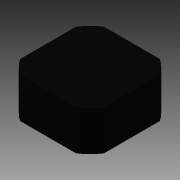
# Autodesk Inventor part: stepper_middle
Saved by Autodesk Inventor 2013 (Build 170138000, 138)
## iProperties
Shininess: 20.0
Created: 2011-05-14
Part Number: stepper_middle
Document SubType Name: Modeling
Designer: Noa Izumi
Material: Default
Density: 1 g/cm^3
Density: 0.0
Volumn: 0.0
Area: 0.0
PropertySet Name: Model Information
Control State: 0
Master: False
Checked Out: False
Author: Noa Izumi
Autodesk Inventor part; units mm, degrees
ref_plane "YZ Plane" through (0, 0, 0) normal (1, 0, 0) x (0, 1, 0)
ref_plane "XZ Plane" through (0, 0, 0) normal (0, 1, 0) x (-1, 0, 0)
ref_plane "XY Plane" through (0, 0, 0) normal (0, 0, 1) x (1, 0, 0)
sketch "Sketch1" plane through (0, 0, 0) normal (0, 0, 1) x (1, 0, 0)
  line L0 (6.9799, 0) -> (35.0201, 0)
  line L1 (42, 6.9799) -> (42, 35.0201)
  line L2 (35.0201, 42) -> (6.9799, 42)
  line L3 (0, 35.0201) -> (0, 6.9799)
  arc A0 (42, 35.0201) -> (35.0201, 42) centre (21, 21) ccw
  arc A1 (35.0201, 0) -> (42, 6.9799) centre (21, 21) ccw
  arc A2 (6.9799, 42) -> (0, 35.0201) centre (21, 21) ccw
  arc A3 (0, 6.9799) -> (6.9799, 0) centre (21, 21) ccw
  dimension "d11" = 42
  dimension "d12" = 42
  constraints: 8 end point, 8 point on circle, 4 centre point, 2 parallel, 1 horizontal, 1 perpendicular
  measures "d11" distance between parallel lines of L0 L2
  measures "d12" distance between parallel lines of L1 L3
extrude "Extrusion1" add sketch "Sketch1" along normal blind 20
